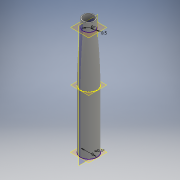
# Autodesk Inventor part: Hand
Saved by Autodesk Inventor 2016 (Build 200138000, 138)
## iProperties
Created: 2015-12-24
Part Number: Hand
Material: Generic
Document SubType Name: Modeling
Designer: gregg
Density: 1 g/cm^3
Appearance: Default
Author: gregg
Autodesk Inventor part; units mm, degrees
ref_plane "YZ Plane" through (0, 0, 0) normal (1, 0, 0) x (0, 1, 0)
ref_plane "XZ Plane" through (0, 0, 0) normal (0, 1, 0) x (-1, 0, 0)
sketch "Sketch1" plane through (0, 0, 0) normal (0, 0, 1) x (1, 0, 0)
  circle A0 centre (0, 0) radius 4.5
  circle A1 centre (0, 0) radius 5
  line L0 (0, 0) -> (0, -5)
  dimension "d0" = 9
  dimension "d1" = 0.5
  constraints: 2 coincident, 2 end point, 1 centre point, 1 vertical, 1 vertical alignment, 2 other
  measures "d0" diameter of A0
ref_plane "Work Plane1" through (0, 0, 35) normal (0, 0, 1) x (1, 0, 0)
ref_plane "Work Plane2" through (0, 0, 65) normal (0, 0, 1) x (1, 0, 0)
sketch "Sketch3" plane through (0, 0, 65) normal (0, 0, 1) x (1, 0, 0)
  circle A0 centre (0, 0) radius 3
  circle A1 centre (0, 0) radius 3.5
  line L0 (0, 0) -> (0, -3.5)
  dimension "d4" = 0.5
  dimension "d5" = 6
  constraints: 2 coincident, 2 end point, 1 centre point, 1 vertical, 1 vertical alignment, 2 other
  measures "d5" diameter of A0
sketch "Sketch2" plane through (0, 0, 35) normal (0, 0, 1) x (1, 0, 0)
  circle A0 centre (0, 0) radius 5 projected
  circle A1 centre (0, 0) radius 4.5 projected
  line L0 (0, 0) -> (0, -5)
  constraints: 2 end point, 1 vertical, 1 vertical alignment, 1 other
ref_plane "Work Plane3" through (0, 0, 0) normal (-1, 0, 0) x (0, -1, 0)
sketch "Sketch4" plane through (0, 0, 0) normal (-1, 0, 0) x (0, -1, 0)
  line L0 (5, 35) -> (5, 0)
  line L1 (5, 0) -> (4.5, 0)
  line L2 (4.5, 0) -> (4.5, 35)
  arc A0 (5, 35) -> (3.5, 65) centre (-295.75, 35) ccw
  line L3 (5, 0) -> (-5, 0) projected
  line L4 (4.5, 0) -> (-4.5, 0) projected
  line L5 (0, 0) -> (5, 0) projected
  line L6 (5, 35) -> (-5, 35) projected
  line L7 (0, 35) -> (5, 35) projected
  line L8 (4.5, 35) -> (-4.5, 35) projected
  line L9 (0, 65) -> (3.5, 65) projected
  line L10 (3.5, 65) -> (-3.5, 65) projected
  line L11 (3, 65) -> (-3, 65) projected
  line L12 (3.5, 65) -> (3, 65)
  arc A1 (4.5, 35) -> (3, 65) centre (-296.25, 35) ccw
  line L13 (0, 65) -> (0, 0)
  constraints: 10 end point, 4 point on circle, 2 centre point, 2 perpendicular, 2 tangent, 1 parallel
revolve "Revolution2" add sketch "Sketch4" angle 360 about axis through (0, 0, 65) along (0, 0, -1) contours L6 A1 L9 A0 | L0 L1 L2 L6
sketch "Sketch5" plane through (0, 0, 65) normal (0, 0, 1) x (1, 0, 0)
  circle A0 centre (0, 0) radius 3.5
  circle A1 centre (0, 0) radius 2
  circle A2 centre (0, 0) radius 3 projected
  dimension "d21" = 4
  constraints: 2 centre point, 2 coincident
  measures "d21" diameter of A1
extrude "Extrusion1" add sketch "Sketch5" along normal blind 5 contours A0
body "Solid3"
